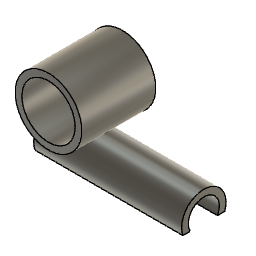
3-Attache_moteurs_sans_reducteur (Autodesk Fusion 360 design; units mm, degrees)
Autodesk Fusion 360 part; units mm, degrees
note: some values were not read from the file. Chosen so that the rebuilt part matches the saved one: which face or edge a step refers to. Set by a fixed rule: which sketch regions a step uses.
sketch "Sketch1" plane through (0, 0, 0) normal (0, 1, 0) x (1, 0, 0)
  circle A0 centre (0, 0) radius 3.6
  circle A1 centre (0, 0) radius 4.5
  dimension "d1" = 7.2
  dimension "d2" = 9
  constraint coincident A0.centre A1.centre
  constraint concentric A0 A1
  measures "d1" diameter of A0
  measures "d2" diameter of A1
extrude "Extrude1" add sketch "Sketch1" along normal mid plane 10
sketch "Sketch2" plane through (0, 0, 0) normal (1, 0, 0) x (0, 1, 0)
  circle A0 centre (0, -6.6) radius 2.1
  circle A1 centre (0, -6.6) radius 3
  dimension "d17" = 4.2
  dimension "d18" = 6
  dimension "d19" = 6.6
  constraint concentric A0 A1
  measures "d17" diameter of A0
  measures "d18" diameter of A1
  measures "d19" distance of origin A0.centre
extrude "Extrusion5" add sketch "Sketch2" along normal blind 16 and the other way blind 4
sketch "Esquisse4" plane through (16, 0, 0) normal (1, 0, 0) x (0, 1, 0)
  circle A0 centre (0, -6.6) radius 2.1
  circle A1 centre (0, -6.6) radius 3
  line L0 (-4, -7.6) -> (4, -7.6)
  line L1 (4, -7.6) -> (4, -10.6)
  line L2 (4, -10.6) -> (-4, -10.6)
  line L3 (-4, -10.6) -> (-4, -7.6)
  dimension "d24" = 1
  dimension "d25" = 3
  constraint horizontal L0
  constraint vertical L1
  constraint horizontal L2
  constraint vertical L3
  measures "d24" distance of A0.centre L0
  measures "d25" distance of L0.end L1.end
extrude "Extrusion6" cut sketch "Esquisse4" against normal blind 22 contours A0 L0 | A0 A1 L0 | A1 L0 L1 L2 L3 picked at (0.3668, -7.9106) picked at (-2.3087, -7.988)
extrude "Extrude2" [suppressed]
extrude "Extrude3" [suppressed]
fillet "Fillet1" [suppressed]
fillet "Fillet2" [suppressed]
sketch "Sketch3" plane through (18, 0, 0) normal (1, 0, 0) x (0, 1, 0)
  circle A0 centre (0, 0) radius 2.6
  circle A1 centre (0, 0) radius 3.5
  line L0 (-5.5, -3.5) -> (5.3771, -3.5)
  line L1 (5.3771, -3.5) -> (5.3771, -4.7708)
  line L2 (5.3771, -4.7708) -> (-5.5, -4.7708)
  line L3 (-5.5, -4.7708) -> (-5.5, -3.5)
  constraint horizontal L0
  constraint vertical L1
  constraint horizontal L2
  constraint vertical L3
extrude "Extrude4" [suppressed]
